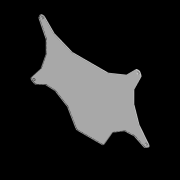
# Autodesk Inventor part: DriverManifoldBase
Saved by Autodesk Inventor 2020 (Build 240168000, 168)
## iProperties
Created: 2020-12-05
Part Number: DriverManifoldBase
Material: Generic
Document SubType Name: Sheet Metal
Designer: valer
Density: 1 g/cm^3
Sheet Metal Rule: Default
Appearance: Default
Author: valer
Autodesk Inventor part; units mm, degrees
ref_plane "YZ Plane" through (0, 0, 0) normal (1, 0, 0) x (0, 1, 0)
ref_plane "XZ Plane" through (0, 0, 0) normal (0, 1, 0) x (-1, 0, 0)
ref_plane "XY Plane" through (0, 0, 0) normal (0, 0, 1) x (1, 0, 0)
sketch "Sketch1" plane through (0, 0, 0) normal (0, 0, 1) x (1, 0, 0)
  circle A0 centre (-403.2911, 84.3356) radius 3.175
  line L0 (-234.0613, -196.9859) -> (-234.0613, 203.2) construction
  line L1 (-414.7517, 79.7013) -> (-409.2875, 93.2256)
  line L2 (-409.2875, 93.2256) -> (-397.0686, 93.2256)
  line L3 (-397.0686, 93.2256) -> (-361.1475, 57.3046)
  line L4 (-361.1475, 57.3046) -> (-297.5613, 31.6141)
  line L5 (-297.5613, 31.6141) -> (-234.0613, 31.6141)
  line L6 (-414.7517, 79.7013) -> (-388.7709, 26.4328)
  line L7 (-388.7709, 26.4328) -> (-388.7709, -19.2872)
  line L8 (-388.7709, -19.2872) -> (-406.9636, -72.1228)
  line L9 (-406.9636, -72.1228) -> (-446.0581, -122.1615)
  line L10 (-446.0581, -122.1615) -> (-427.2965, -131.1739)
  line L11 (-427.2965, -131.1739) -> (-390.6155, -113.6779)
  line L12 (-390.6155, -113.6779) -> (-356.7952, -115.4504)
  line L13 (-356.7952, -115.4504) -> (-313.4811, -141.9933)
  line L14 (-313.4811, -141.9933) -> (-281.7311, -196.9859)
  line L15 (-281.7311, -196.9859) -> (-234.0613, -196.9859)
  circle A1 centre (-432.2524, -118.9308) radius 3.175
  circle A2 centre (-64.8315, 84.3356) radius 3.175
  line L16 (-53.3709, 79.7013) -> (-58.8351, 93.2256)
  line L17 (-58.8351, 93.2256) -> (-71.054, 93.2256)
  line L18 (-71.054, 93.2256) -> (-106.975, 57.3046)
  line L19 (-106.975, 57.3046) -> (-170.5613, 31.6141)
  line L20 (-170.5613, 31.6141) -> (-234.0613, 31.6141)
  line L21 (-53.3709, 79.7013) -> (-79.3517, 26.4328)
  line L22 (-79.3517, 26.4328) -> (-79.3517, -19.2872)
  line L23 (-79.3517, -19.2872) -> (-61.1589, -72.1228)
  line L24 (-61.1589, -72.1228) -> (-22.0644, -122.1615)
  line L25 (-22.0644, -122.1615) -> (-40.826, -131.1739)
  line L26 (-40.826, -131.1739) -> (-77.5071, -113.6779)
  line L27 (-77.5071, -113.6779) -> (-111.3273, -115.4504)
  line L28 (-111.3273, -115.4504) -> (-154.6415, -141.9933)
  line L29 (-154.6415, -141.9933) -> (-186.3915, -196.9859)
  line L30 (-186.3915, -196.9859) -> (-234.0613, -196.9859)
  circle A3 centre (-35.8701, -118.9308) radius 3.175
  dimension "d0" = 63.5
  dimension "d1" = 158
  dimension "d2" = 68.58
  dimension "d3" = 157
  dimension "d4" = 50.8
  dimension "d5" = 112
  dimension "d6" = 8.89
  dimension "d7" = 8.89
  dimension "d8" = 132
  dimension "d9" = 59.2667
  dimension "d10" = 154
  dimension "d11" = 45.72
  dimension "d12" = 161
  dimension "d13" = 161
  dimension "d14" = 55.88
  dimension "d15" = 8.89
  dimension "d16" = 8.89
  dimension "d17" = 63.5
  dimension "d18" = 228.6
  dimension "d19" = 120
  dimension "d20" = 63.5
  dimension "d21" = 151.5
  dimension "d22" = 50.8
  dimension "d23" = 151.5
  dimension "d24" = 33.8667
  dimension "d25" = 151.5
  dimension "d26" = 40.64
  dimension "d27" = 20.8139
  measures "d0" distance of L4.end L5.end
  measures "d1" angle of L5 L4
  measures "d2" distance of L3.end L4.end
  measures "d3" angle of L4 L3
  measures "d4" distance of L2.end L3.end
  measures "d5" angle of L2 L1
  measures "d6" distance from line of L2 A0.centre
  measures "d7" distance from line of L1 A0.centre
  measures "d8" angle of L1 L6
  measures "d9" distance of L1.start L6.end
  measures "d10" angle of L6 L7
  measures "d11" distance of L6.end L7.end
  measures "d12" angle of L7 L8
  measures "d13" angle of L9 L8
  measures "d14" distance of L7.end L8.end
  measures "d15" distance from line of L10 A1.centre
  measures "d16" distance from line of L9 A1.centre
  measures "d17" distance of L8.end L9.end
  measures "d18" distance between parallel lines of L5 L15
  measures "d19" angle of L15 L14
  measures "d20" distance of L13.end L14.end
  measures "d21" angle of L14 L13
  measures "d22" distance of L12.end L13.end
  measures "d23" angle of L13 L12
  measures "d24" distance of L11.end L12.end
  measures "d25" angle of L12 L11
  measures "d26" distance of L10.end L11.end
  measures "d27" distance of L9.end L10.end
extrude "Plate1" add sketch "Sketch1" along normal blind 3.048
fillet "Fillet1" radius 6.35 28 edges at (-446.0581, -122.1615, 1.524) (-427.2965, -131.1739, 1.524) (-406.9636, -72.1228, 1.524) (-390.6155, -113.6779, 1.524) (-388.7709, -19.2872, 1.524) (-388.7709, 26.4328, 1.524) (-414.7517, 79.7013, 1.524) (-409.2875, 93.2256, 1.524) (-313.4811, -141.9933, 1.524) (-281.7311, -196.9859, 1.524) (-186.3915, -196.9859, 1.524) (-154.6415, -141.9933, 1.524) (-111.3273, -115.4504, 1.524) (-77.5071, -113.6779, 1.524) (-40.826, -131.1739, 1.524) (-22.0644, -122.1615, 1.524) (-61.1589, -72.1228, 1.524) (-79.3517, -19.2872, 1.524) (-79.3517, 26.4328, 1.524) (-53.3709, 79.7013, 1.524) (-58.8351, 93.2256, 1.524) (-71.054, 93.2256, 1.524) (-106.975, 57.3046, 1.524) (-170.5613, 31.6141, 1.524) (-297.5613, 31.6141, 1.524) (-361.1475, 57.3046, 1.524) (-397.0686, 93.2256, 1.524) (-356.7952, -115.4504, 1.524)
equation "\"d28\" = Thickness"
equation "\"BendRadius\" = Thickness"
equation "\"BendReliefWidth\" = Thickness"
equation "\"BendReliefDepth\" = 0.5 * Thickness"
equation "\"CornerReliefSize\" = 4 * Thickness"
equation "\"MinimumRemnant\" = 2 * Thickness"
equation "\"TransitionRadius\" = BendRadius"
equation "\"JacobiRadiusSize\" = BendRadius"
equation "\"GapSize\" = Thickness"
equation "\"Thickness\" = 3.048"
body "Solid1"
